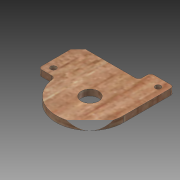
# Autodesk Inventor part: p6
Saved by Autodesk Inventor 2015 (Build 190159000, 159)
## iProperties
Created: 2016-02-03
Part Number: p6
Material: Generic
Document SubType Name: Modeling
Designer: david
Density: 1 g/cm^3
Appearance: Birch - Natural Polished
Mass: 6.40214 g
Surface Area: 43.8659 cm^2
Volume: 6.40214 cm^3
Author: david
Autodesk Inventor part; units mm, degrees
ref_plane "YZ Plane" through (0, 0, 0) normal (1, 0, 0) x (0, 1, 0)
ref_plane "XZ Plane" through (0, 0, 0) normal (0, 1, 0) x (-1, 0, 0)
ref_plane "XY Plane" through (0, 0, 0) normal (0, 0, 1) x (1, 0, 0)
sketch "Sketch1" plane through (0, 0, 0) normal (0, 0, 1) x (1, 0, 0)
  circle A0 centre (24.9974, -44.3363) radius 20
  line L0 (44.9974, -44.3363) -> (30.9974, -44.3363)
  line L1 (30.9974, -44.3363) -> (30.9974, -14.3363)
  line L2 (30.9974, -14.3363) -> (44.9974, -14.3363)
  line L3 (44.9974, -14.3363) -> (44.9974, -44.3363)
  line L4 (30.9974, -21.407) -> (-4.9442, -21.407)
  line L5 (-4.9442, -21.407) -> (-4.9442, -45.1154)
  line L6 (-4.9442, -45.1154) -> (30.9974, -45.1154)
  line L7 (30.9974, -45.1154) -> (30.9974, -21.407)
  point P0 (0, 0)
  dimension "d0" = 40
  dimension "d1" = 14
  dimension "d2" = 30
  constraints: 16 end point, 4 parallel, 2 horizontal, 2 perpendicular, 1 horizontal alignment, 1 point on line, 2 other
  measures "d1" distance of L1.end L2.end
  measures "d2" distance of L0.end L1.end
extrude "Extrusion1" add sketch "Sketch1" along normal blind 3.6
sketch "Sketch2" plane through (0, 0, 3.6) normal (0, 0, 1) x (1, 0, 0)
  arc A0 (5.0125, -45.1154) -> (44.9974, -44.3363) centre (24.9974, -44.3363) ccw projected
  circle A1 centre (24.9974, -44.3363) radius 5.15
  circle A2 centre (-0.4442, -40.6154) radius 1.625
  line L0 (-4.9442, -21.407) -> (-4.9442, -45.1154) projected
  line L1 (-4.9442, -45.1154) -> (5.0125, -45.1154) projected
  circle A3 centre (40.4974, -19.3363) radius 1.625
  line L2 (44.9974, -44.3363) -> (44.9974, -14.3363) projected
  point P0 (0, 0)
  dimension "d5" = 10.3
  dimension "d6" = 3.25
  dimension "d9" = 4.5
  dimension "d10" = 4.5
  dimension "d11" = 3.25
  dimension "d12" = 4.5
  dimension "d13" = 25
  constraints: 3 centre point, 1 coincident
  measures "d5" diameter of A1
  measures "d6" diameter of A2
  measures "d9" distance from line of L0 A2.centre
  measures "d10" distance from line of L1 A2.centre
  measures "d11" diameter of A3
  measures "d12" distance from line of L2 A3.centre
  measures "d13" vertical distance of A0.centre A3.centre
extrude "Extrusion2" cut sketch "Sketch2" against normal blind 20
fillet "Fillet1" radius 2 6 edges at (44.9974, -14.3363, 1.8) (-4.9442, -45.1154, 1.8) (30.9974, -14.3363, 1.8) (-4.9442, -21.407, 1.8) (30.9974, -21.407, 1.8) (5.0125, -45.1154, 1.8)
body "Solid1"
